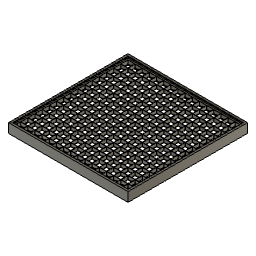
LED matrix v11 (Autodesk Fusion 360 design; units mm, degrees)
Autodesk Fusion 360 part; units mm, degrees
sketch "quad" plane through (0, 0, 0) normal (0, 0, 1) x (1, 0, 0)
  line L0 (0, 0) -> (10, 0)
  line L1 (10, 0) -> (10, 10)
  line L2 (10, 10) -> (0, 10)
  line L3 (0, 10) -> (0, 0)
  line L4 (9.75, 0.25) -> (9.75, 9.75)
  line L5 (9.75, 9.75) -> (0.25, 9.75)
  line L6 (0.25, 9.75) -> (0.25, 0.25)
  line L7 (0.25, 0.25) -> (9.75, 0.25)
  dimension "d1" = 10
  dimension "d2" = 10
  dimension "d3" = -0.25
  constraint horizontal L0
  constraint vertical L1
  constraint horizontal L2
  constraint vertical L3
  constraint coincident L0.start L3.end
  measures "d1" distance of L0.start L0.end
  measures "d2" distance of L0.start L2.end
extrude "Extrude1" add sketch "quad" along normal blind 5 makes body 1
sketch "hole" plane through (0, 0, 0) normal (0, 1, 0) x (1, 0, 0)
  line L0 (4.3, 0) -> (7.3, 0)
  line L1 (7.3, 0) -> (7.3, -0.5)
  line L2 (7, -0.8) -> (4.6, -0.8)
  line L3 (4.3, -0.5) -> (4.3, 0)
  arc A0 (4.3, -0.5) -> (4.6, -0.8) centre (4.6, -0.5) ccw
  arc A1 (7, -0.8) -> (7.3, -0.5) centre (7, -0.5) ccw
  point P0 (4.3, -0.8)
  point P1 (10, 0)
  dimension "d6" = 3
  dimension "d7" = 0.8
  dimension "d8" = 2.7
  dimension "d11" = 0.3
  dimension "d12" = 0.3
  constraint horizontal L0
  constraint vertical L1
  constraint horizontal L2
  constraint vertical L3
  constraint coincident P0 L2
  constraint coincident P0 L3
  constraint tangent L2 A0
  constraint tangent L3 A0
  constraint tangent L1 A1
  constraint tangent L2 A1
  measures "d6" distance of L0.start L0.end
  measures "d7" distance of L0.start P0
  measures "d8" distance of L0.end P1
  measures "d11" radius of A0
  measures "d12" radius of A1
extrude "Extrude2" cut sketch "hole" along normal blind 10 bodies 1
sketch "lid" plane through (0, 0, 5) normal (0, 0, 1) x (-1, 0, 0)
  line L0 (-9.75, -0.25) -> (-0.25, -0.25)
  line L1 (-0.25, -0.25) -> (-0.25, -9.75)
  line L2 (-0.25, -9.75) -> (-9.75, -9.75)
  line L3 (-9.75, -9.75) -> (-9.75, -0.25)
  line L4 (0, -10) -> (0, 0)
  line L5 (0, 0) -> (-10, 0)
  line L6 (-10, 0) -> (-10, -10)
  line L7 (-10, -10) -> (0, -10)
  line L8 (0, 0) -> (-10, 0)
  line L9 (-10, 0) -> (-10, -10)
  line L10 (-10, -10) -> (0, -10)
  line L11 (0, -10) -> (0, 0)
  constraint horizontal L8
  constraint vertical L9
  constraint horizontal L10
  constraint vertical L11
  constraint coincident L6.end L7.start
  constraint coincident L4.end L5.start
extrude "Extrude3" add sketch "lid" along normal blind 0.2 separate body contours L0 L1 L2 L3 | L4 L5 L6 L7 L8 L9 L10 L11 makes body 2
pattern_linear "R-Pattern1" count 16 spacing 10 along (0, 1, 0) count 16 spacing 10 along (1, 0, 0) of bodies 1 makes body 3 at (0, 16.6667, 1.6667) makes body 4 at (0, 26.6667, 1.6667) makes body 5 at (10, 6.6667, 1.6667) makes body 6 at (10.25, 16.5833, 1.6667) makes body 7 at (10.25, 26.5833, 1.6667) makes body 8 at (24.8667, 0, 3.6) makes body 9 at (20.25, 16.5833, 1.6667) makes body 10 at (20.25, 26.5833, 1.6667) makes body 11 at (0, 36.6667, 1.6667) makes body 12 at (0, 46.6667, 1.6667) makes body 13 at (0, 56.6667, 1.6667) makes body 14 at (0, 66.6667, 1.6667) makes body 15 at (0, 76.6667, 1.6667) makes body 16 at (0, 86.6667, 1.6667) makes body 17 at (0, 96.6667, 1.6667) makes body 18 at (0, 106.6667, 1.6667) makes body 19 at (0, 116.6667, 1.6667) makes body 20 at (0, 126.6667, 1.6667) makes body 21 at (0, 136.6667, 1.6667) makes body 22 at (0, 146.6667, 1.6667) makes body 23 at (0, 156.6667, 1.6667) makes body 24 at (10.25, 36.5833, 1.6667) makes body 25 at (10.25, 46.5833, 1.6667) makes body 26 at (10.25, 56.5833, 1.6667) makes body 27 at (10.25, 66.5833, 1.6667) makes body 28 at (10.25, 76.5833, 1.6667) makes body 29 at (10.25, 86.5833, 1.6667) makes body 30 at (10.25, 96.5833, 1.6667) makes body 31 at (10.25, 106.5833, 1.6667) makes body 32 at (10.25, 116.5833, 1.6667) makes body 33 at (10.25, 126.5833, 1.6667) makes body 34 at (10.25, 136.5833, 1.6667) makes body 35 at (10.25, 146.5833, 1.6667) makes body 36 at (14.8667, 160, 3.6) makes body 37 at (20.25, 36.5833, 1.6667) makes body 38 at (20.25, 46.5833, 1.6667) makes body 39 at (20.25, 56.5833, 1.6667) makes body 40 at (20.25, 66.5833, 1.6667) makes body 41 at (20.25, 76.5833, 1.6667) makes body 42 at (20.25, 86.5833, 1.6667) makes body 43 at (20.25, 96.5833, 1.6667) makes body 44 at (20.25, 106.5833, 1.6667) makes body 45 at (20.25, 116.5833, 1.6667) makes body 46 at (20.25, 126.5833, 1.6667) makes body 47 at (20.25, 136.5833, 1.6667) makes body 48 at (20.25, 146.5833, 1.6667) makes body 49 at (24.8667, 160, 3.6) makes body 50 at (34.8667, 0, 3.6) makes body 51 at (30.25, 16.5833, 1.6667) makes body 52 at (30.25, 26.5833, 1.6667) makes body 53 at (30.25, 36.5833, 1.6667) makes body 54 at (30.25, 46.5833, 1.6667) makes body 55 at (30.25, 56.5833, 1.6667) makes body 56 at (30.25, 66.5833, 1.6667) makes body 57 at (30.25, 76.5833, 1.6667) makes body 58 at (30.25, 86.5833, 1.6667) makes body 59 at (30.25, 96.5833, 1.6667) makes body 60 at (30.25, 106.5833, 1.6667) makes body 61 at (30.25, 116.5833, 1.6667) makes body 62 at (30.25, 126.5833, 1.6667) makes body 63 at (30.25, 136.5833, 1.6667) makes body 64 at (30.25, 146.5833, 1.6667) makes body 65 at (34.8667, 160, 3.6) makes body 66 at (44.8667, 0, 3.6) makes body 67 at (40.25, 16.5833, 1.6667) makes body 68 at (40.25, 26.5833, 1.6667) makes body 69 at (40.25, 36.5833, 1.6667) makes body 70 at (40.25, 46.5833, 1.6667) makes body 71 at (40.25, 56.5833, 1.6667) makes body 72 at (40.25, 66.5833, 1.6667) makes body 73 at (40.25, 76.5833, 1.6667) makes body 74 at (40.25, 86.5833, 1.6667) makes body 75 at (40.25, 96.5833, 1.6667) makes body 76 at (40.25, 106.5833, 1.6667) makes body 77 at (40.25, 116.5833, 1.6667) makes body 78 at (40.25, 126.5833, 1.6667) makes body 79 at (40.25, 136.5833, 1.6667) makes body 80 at (40.25, 146.5833, 1.6667) makes body 81 at (44.8667, 160, 3.6) makes body 82 at (54.8667, 0, 3.6) makes body 83 at (50.25, 16.5833, 1.6667) makes body 84 at (50.25, 26.5833, 1.6667) makes body 85 at (50.25, 36.5833, 1.6667) makes body 86 at (50.25, 46.5833, 1.6667) makes body 87 at (50.25, 56.5833, 1.6667) makes body 88 at (50.25, 66.5833, 1.6667) makes body 89 at (50.25, 76.5833, 1.6667) makes body 90 at (50.25, 86.5833, 1.6667) makes body 91 at (50.25, 96.5833, 1.6667) makes body 92 at (50.25, 106.5833, 1.6667) makes body 93 at (50.25, 116.5833, 1.6667) makes body 94 at (50.25, 126.5833, 1.6667) makes body 95 at (50.25, 136.5833, 1.6667) makes body 96 at (50.25, 146.5833, 1.6667) makes body 97 at (54.8667, 160, 3.6) makes body 98 at (64.8667, 0, 3.6) makes body 99 at (60.25, 16.5833, 1.6667) makes body 100 at (60.25, 26.5833, 1.6667) makes body 101 at (60.25, 36.5833, 1.6667) makes body 102 at (60.25, 46.5833, 1.6667) makes body 103 at (60.25, 56.5833, 1.6667) makes body 104 at (60.25, 66.5833, 1.6667) makes body 105 at (60.25, 76.5833, 1.6667) makes body 106 at (60.25, 86.5833, 1.6667) makes body 107 at (60.25, 96.5833, 1.6667) makes body 108 at (60.25, 106.5833, 1.6667) makes body 109 at (60.25, 116.5833, 1.6667) makes body 110 at (60.25, 126.5833, 1.6667) makes body 111 at (60.25, 136.5833, 1.6667) makes body 112 at (60.25, 146.5833, 1.6667) makes body 113 at (64.8667, 160, 3.6) makes body 114 at (74.8667, 0, 3.6) makes body 115 at (70.25, 16.5833, 1.6667) makes body 116 at (70.25, 26.5833, 1.6667) makes body 117 at (70.25, 36.5833, 1.6667) makes body 118 at (70.25, 46.5833, 1.6667) makes body 119 at (70.25, 56.5833, 1.6667) makes body 120 at (70.25, 66.5833, 1.6667) makes body 121 at (70.25, 76.5833, 1.6667) makes body 122 at (70.25, 86.5833, 1.6667) makes body 123 at (70.25, 96.5833, 1.6667) makes body 124 at (70.25, 106.5833, 1.6667) makes body 125 at (70.25, 116.5833, 1.6667) makes body 126 at (70.25, 126.5833, 1.6667) makes body 127 at (70.25, 136.5833, 1.6667) makes body 128 at (70.25, 146.5833, 1.6667) makes body 129 at (74.8667, 160, 3.6) makes body 130 at (84.8667, 0, 3.6) makes body 131 at (80.25, 16.5833, 1.6667) makes body 132 at (80.25, 26.5833, 1.6667) makes body 133 at (80.25, 36.5833, 1.6667) makes body 134 at (80.25, 46.5833, 1.6667) makes body 135 at (80.25, 56.5833, 1.6667) makes body 136 at (80.25, 66.5833, 1.6667) makes body 137 at (80.25, 76.5833, 1.6667) makes body 138 at (80.25, 86.5833, 1.6667) makes body 139 at (80.25, 96.5833, 1.6667) makes body 140 at (80.25, 106.5833, 1.6667) makes body 141 at (80.25, 116.5833, 1.6667) makes body 142 at (80.25, 126.5833, 1.6667) makes body 143 at (80.25, 136.5833, 1.6667) makes body 144 at (80.25, 146.5833, 1.6667) makes body 145 at (84.8667, 160, 3.6) makes body 146 at (94.8667, 0, 3.6) makes body 147 at (90.25, 16.5833, 1.6667) makes body 148 at (90.25, 26.5833, 1.6667) makes body 149 at (90.25, 36.5833, 1.6667) makes body 150 at (90.25, 46.5833, 1.6667) makes body 151 at (90.25, 56.5833, 1.6667) makes body 152 at (90.25, 66.5833, 1.6667) makes body 153 at (90.25, 76.5833, 1.6667) makes body 154 at (90.25, 86.5833, 1.6667) makes body 155 at (90.25, 96.5833, 1.6667) makes body 156 at (90.25, 106.5833, 1.6667) makes body 157 at (90.25, 116.5833, 1.6667) makes body 158 at (90.25, 126.5833, 1.6667) makes body 159 at (90.25, 136.5833, 1.6667) makes body 160 at (90.25, 146.5833, 1.6667) makes body 161 at (94.8667, 160, 3.6) makes body 162 at (104.8667, 0, 3.6) makes body 163 at (100.25, 16.5833, 1.6667) makes body 164 at (100.25, 26.5833, 1.6667) makes body 165 at (100.25, 36.5833, 1.6667) makes body 166 at (100.25, 46.5833, 1.6667) makes body 167 at (100.25, 56.5833, 1.6667) makes body 168 at (100.25, 66.5833, 1.6667) makes body 169 at (100.25, 76.5833, 1.6667) makes body 170 at (100.25, 86.5833, 1.6667) makes body 171 at (100.25, 96.5833, 1.6667) makes body 172 at (100.25, 106.5833, 1.6667) makes body 173 at (100.25, 116.5833, 1.6667) makes body 174 at (100.25, 126.5833, 1.6667) makes body 175 at (100.25, 136.5833, 1.6667) makes body 176 at (100.25, 146.5833, 1.6667) makes body 177 at (104.8667, 160, 3.6) makes body 178 at (114.8667, 0, 3.6) makes body 179 at (110.25, 16.5833, 1.6667) makes body 180 at (110.25, 26.5833, 1.6667) makes body 181 at (110.25, 36.5833, 1.6667) makes body 182 at (110.25, 46.5833, 1.6667) makes body 183 at (110.25, 56.5833, 1.6667) makes body 184 at (110.25, 66.5833, 1.6667) makes body 185 at (110.25, 76.5833, 1.6667) makes body 186 at (110.25, 86.5833, 1.6667) makes body 187 at (110.25, 96.5833, 1.6667) makes body 188 at (110.25, 106.5833, 1.6667) makes body 189 at (110.25, 116.5833, 1.6667) makes body 190 at (110.25, 126.5833, 1.6667) makes body 191 at (110.25, 136.5833, 1.6667) makes body 192 at (110.25, 146.5833, 1.6667) makes body 193 at (114.8667, 160, 3.6) makes body 194 at (124.8667, 0, 3.6) makes body 195 at (120.25, 16.5833, 1.6667) makes body 196 at (120.25, 26.5833, 1.6667) makes body 197 at (120.25, 36.5833, 1.6667) makes body 198 at (120.25, 46.5833, 1.6667) makes body 199 at (120.25, 56.5833, 1.6667) makes body 200 at (120.25, 66.5833, 1.6667) makes body 201 at (120.25, 76.5833, 1.6667) makes body 202 at (120.25, 86.5833, 1.6667) makes body 203 at (120.25, 96.5833, 1.6667) makes body 204 at (120.25, 106.5833, 1.6667) makes body 205 at (120.25, 116.5833, 1.6667) makes body 206 at (120.25, 126.5833, 1.6667) makes body 207 at (120.25, 136.5833, 1.6667) makes body 208 at (120.25, 146.5833, 1.6667) makes body 209 at (124.8667, 160, 3.6) makes body 210 at (134.8667, 0, 3.6) makes body 211 at (130.25, 16.5833, 1.6667) makes body 212 at (130.25, 26.5833, 1.6667) makes body 213 at (130.25, 36.5833, 1.6667) makes body 214 at (130.25, 46.5833, 1.6667) makes body 215 at (130.25, 56.5833, 1.6667) makes body 216 at (130.25, 66.5833, 1.6667) makes body 217 at (130.25, 76.5833, 1.6667) makes body 218 at (130.25, 86.5833, 1.6667) makes body 219 at (130.25, 96.5833, 1.6667) makes body 220 at (130.25, 106.5833, 1.6667) makes body 221 at (130.25, 116.5833, 1.6667) makes body 222 at (130.25, 126.5833, 1.6667) makes body 223 at (130.25, 136.5833, 1.6667) makes body 224 at (130.25, 146.5833, 1.6667) makes body 225 at (134.8667, 160, 3.6) makes body 226 at (144.8667, 0, 3.6) makes body 227 at (140.25, 16.5833, 1.6667) makes body 228 at (140.25, 26.5833, 1.6667) makes body 229 at (140.25, 36.5833, 1.6667) makes body 230 at (140.25, 46.5833, 1.6667) makes body 231 at (140.25, 56.5833, 1.6667) makes body 232 at (140.25, 66.5833, 1.6667) makes body 233 at (140.25, 76.5833, 1.6667) makes body 234 at (140.25, 86.5833, 1.6667) makes body 235 at (140.25, 96.5833, 1.6667) makes body 236 at (140.25, 106.5833, 1.6667) makes body 237 at (140.25, 116.5833, 1.6667) makes body 238 at (140.25, 126.5833, 1.6667) makes body 239 at (140.25, 136.5833, 1.6667) makes body 240 at (140.25, 146.5833, 1.6667) makes body 241 at (144.8667, 160, 3.6) makes body 242 at (160, 3.3333, 1.6667) makes body 243 at (160, 13.3333, 1.6667) makes body 244 at (160, 23.3333, 1.6667) makes body 245 at (160, 33.3333, 1.6667) makes body 246 at (160, 43.3333, 1.6667) makes body 247 at (160, 53.3333, 1.6667) makes body 248 at (160, 63.3333, 1.6667) makes body 249 at (160, 73.3333, 1.6667) makes body 250 at (160, 83.3333, 1.6667) makes body 251 at (160, 93.3333, 1.6667) makes body 252 at (160, 103.3333, 1.6667) makes body 253 at (160, 113.3333, 1.6667) makes body 254 at (160, 123.3333, 1.6667) makes body 255 at (160, 133.3333, 1.6667) makes body 256 at (160, 143.3333, 1.6667) makes body 257 at (160, 153.3333, 1.6667)
sketch "frame" plane through (0, 0, 0) normal (0, 0, 1) x (1, 0, 0)
  line L0 (0, 0) -> (160, 0)
  line L1 (160, 0) -> (160, 160)
  line L2 (160, 160) -> (0, 160)
  line L3 (0, 160) -> (0, 0)
  line L4 (162, 162) -> (-2, 162)
  line L5 (-2, 162) -> (-2, -2)
  line L6 (-2, -2) -> (162, -2)
  line L7 (162, -2) -> (162, 162)
  line L8 (-3.5, 163.5) -> (-3.5, -3.5)
  line L9 (-3.5, -3.5) -> (163.5, -3.5)
  line L10 (163.5, -3.5) -> (163.5, 163.5)
  line L11 (163.5, 163.5) -> (-3.5, 163.5)
  line L12 (160.5, -0.5) -> (160.5, 160.5)
  line L13 (160.5, 160.5) -> (-0.5, 160.5)
  line L14 (-0.5, 160.5) -> (-0.5, -0.5)
  line L15 (-0.5, -0.5) -> (160.5, -0.5)
  line L16 (162.5, -2.5) -> (162.5, 162.5)
  line L17 (162.5, 162.5) -> (-2.5, 162.5)
  line L18 (-2.5, 162.5) -> (-2.5, -2.5)
  line L19 (-2.5, -2.5) -> (162.5, -2.5)
  dimension "d41" = 160
  dimension "d42" = 160
  dimension "d43" = 2
  dimension "d44" = 3.5
  dimension "d50" = 0.5
  dimension "d59" = 2.5
  constraint horizontal L0
  constraint vertical L1
  constraint horizontal L2
  constraint vertical L3
  constraint coincident L0.start L3.end
  measures "d41" distance of L0.start L0.end
  measures "d42" distance of L0.start L2.end
extrude "Extrude4" add sketch "frame" along normal blind 5 separate body contours L4 L5 L6 L7 | L12 L13 L14 L15 makes body 258
extrude "Extrude9" add sketch "frame" against normal blind 1.5 contours L4 L5 L6 L7 bodies 258
extrude "Extrude6" add sketch "frame" along normal blind 8 and the other way blind 4 separate body contours L8 L9 L10 L11 makes body 259
sketch "lid frame" plane through (0, 0, 8) normal (0, 0, 1) x (-1, 0, 0)
  line L0 (-163.5, -163.5) -> (3.5, -163.5)
  line L1 (3.5, -163.5) -> (3.5, 3.5)
  line L2 (3.5, 3.5) -> (-163.5, 3.5)
  line L3 (-163.5, 3.5) -> (-163.5, -163.5)
  line L4 (-162.5, 2.5) -> (2.5, 2.5)
  line L5 (2.5, 2.5) -> (2.5, -162.5)
  line L6 (2.5, -162.5) -> (-162.5, -162.5)
  line L7 (-162.5, -162.5) -> (-162.5, 2.5)
  line L8 (-160.5, -160.5) -> (-160.5, 0.5)
  line L9 (-160.5, 0.5) -> (0.5, 0.5)
  line L10 (0.5, 0.5) -> (0.5, -160.5)
  line L11 (0.5, -160.5) -> (-160.5, -160.5)
  dimension "d68" = 2
extrude "Extrude7" add sketch "lid frame" along normal blind 1 contours L0 L1 L2 L3 | L4 L5 L6 L7 bodies 259
sketch "PCB hooks" plane through (160.5, 0, 0) normal (-1, 0, 0) x (0, 1, 0)
  line L0 (160, 5) -> (0, 5)
  line L1 (0, 5) -> (0, 0)
  line L2 (0, 0) -> (160, 0)
  line L3 (160, 0) -> (160, 5)
  line L4 (162, -1.5) -> (162, 5)
  line L5 (162, 5) -> (-2, 5)
  line L6 (-2, 5) -> (-2, -1.5)
  line L7 (-2, -1.5) -> (162, -1.5)
  line L8 (-0.5, 0) -> (160.5, 0)
  line L9 (160.5, 0) -> (160.5, 1.5)
  line L10 (160.5, 1.5) -> (-0.5, 1.5)
  line L11 (-0.5, 1.5) -> (-0.5, 0)
  line L12 (3, 1.5) -> (7, 1.5)
  line L13 (7, 1.5) -> (7, 0.5)
  line L14 (7, 0.5) -> (3, 0.5)
  line L15 (3, 0.5) -> (3, 1.5)
  dimension "d53" = 4
  dimension "d54" = 1
  dimension "d55" = 3
  constraint horizontal L12
  constraint vertical L13
  constraint horizontal L14
  constraint vertical L15
  constraint coincident L10 L12.start
  measures "d53" distance of L12.start L12.end
  measures "d54" distance of L12.start L14.end
  measures "d55" distance of L1 L15
extrude "Extrude8" add sketch "PCB hooks" along normal blind 1 separate body contours L10 L12 L13 L14 L15 makes body 260
extrude "Extrude10" add sketch "PCB hooks" against normal blind 1 from surface at 161 separate body contours L10 L12 L13 L14 L15 makes body 261
pattern_linear "R-Pattern2" count 3 spacing 75 along (0, 1, 0) of bodies 261 260 makes body 262 at (160.5, 79.3333, -1.1667) makes body 263 at (160.5, 154.3333, -0.8333) makes body 264 at (-0.5, 79.3333, -1.1667) makes body 265 at (-0.5, 154.3333, -0.8333)
copy_body "CopyPasteBodies2" bodies 260 makes body 266
move_body "Move2" bodies 266 to x (0, 1, 0) y (-1, 0, 0) z (0, 0, 1) at (160, -160, 0)
copy_body "CopyPasteBodies3" bodies 266 makes body 267
move_body "Move3" bodies 267 to x (1, 0, 0) y (0, 1, 0) z (0, 0, 1) at (0, 160, 0)
pattern_linear "R-Pattern3" count 3 spacing 75 along (-1, 0, 0) of bodies 266 267 makes body 268 at (80.6667, 0.5, -1.1667) makes body 269 at (5.6667, 0.5, -1.1667) makes body 270 at (80.6667, 160.5, -1.1667) makes body 271 at (5.6667, 160.5, -1.1667)
hidden bodies 2
equation "h = 5 mm"
equation "d20 = h"
equation "d28 = h + 3 mm"
equation "d48 = -( 160 mm - 3 mm - 4 mm - 3 mm )"
equation "d66 = 160 mm - ( 2 * 3 ) * 1 mm - 4 mm"
named bodies: "box", "lid", "box (1)", "box (2)", "box (3)", "box (4)", "box (5)", "box (6)", "box (7)", "box (8)", "frame grid", "frame lid", "PCB hook 1", "PCB hook (1)", "PCB hook (2)", "box (9)", "box (10)", "box (11)", "box (12)", "box (13)", "box (14)", "box (15)", "box (16)", "box (17)", "box (18)", "box (19)", "box (20)", "box (21)", "box (22)", "box (23)", "box (24)", "box (25)", "box (26)", "box (27)", "box (28)", "box (29)", "box (30)", "box (31)", "box (32)", "box (33)", "box (34)", "box (35)", "box (36)", "box (37)", "box (38)", "box (39)", "box (40)", "box (41)", "box (42)", "box (43)", "box (44)", "box (45)", "box (46)", "box (47)", "box (48)", "box (49)", "box (50)", "box (51)", "box (52)", "box (53)", "box (54)", "box (55)", "box (56)", "box (57)", "box (58)", "box (59)", "box (60)", "box (61)", "box (62)", "box (63)", "box (64)", "box (65)", "box (66)", "box (67)", "box (68)", "box (69)", "box (70)", "box (71)", "box (72)", "box (73)", "box (74)", "box (75)", "box (76)", "box (77)", "box (78)", "box (79)", "box (80)", "box (81)", "box (82)", "box (83)", "box (84)", "box (85)", "box (86)", "box (87)", "box (88)", "box (89)", "box (90)", "box (91)", "box (92)", "box (93)", "box (94)", "box (95)", "box (96)", "box (97)", "box (98)", "box (99)", "box (100)", "box (101)", "box (102)", "box (103)", "box (104)", "box (105)", "box (106)", "box (107)", "box (108)", "box (109)", "box (110)", "box (111)", "box (112)", "box (113)", "box (114)", "box (115)", "box (116)", "box (117)", "box (118)", "box (119)", "box (120)", "box (121)", "box (122)", "box (123)", "box (124)", "box (125)", "box (126)", "box (127)", "box (128)", "box (129)", "box (130)", "box (131)", "box (132)", "box (133)", "box (134)", "box (135)", "box (136)", "box (137)", "box (138)", "box (139)", "box (140)", "box (141)", "box (142)", "box (143)", "box (144)", "box (145)", "box (146)", "box (147)", "box (148)", "box (149)", "box (150)", "box (151)", "box (152)", "box (153)", "box (154)", "box (155)", "box (156)", "box (157)", "box (158)", "box (159)", "box (160)", "box (161)", "box (162)", "box (163)", "box (164)", "box (165)", "box (166)", "box (167)", "box (168)", "box (169)", "box (170)", "box (171)", "box (172)", "box (173)", "box (174)", "box (175)", "box (176)", "box (177)", "box (178)", "box (179)", "box (180)", "box (181)", "box (182)", "box (183)", "box (184)", "box (185)", "box (186)", "box (187)", "box (188)", "box (189)", "box (190)", "box (191)", "box (192)", "box (193)", "box (194)", "box (195)", "box (196)", "box (197)", "box (198)", "box (199)", "box (200)", "box (201)", "box (202)", "box (203)", "box (204)", "box (205)", "box (206)", "box (207)", "box (208)", "box (209)", "box (210)", "box (211)", "box (212)", "box (213)", "box (214)", "box (215)", "box (216)", "box (217)", "box (218)", "box (219)", "box (220)", "box (221)", "box (222)", "box (223)", "box (224)", "box (225)", "box (226)", "box (227)", "box (228)", "box (229)", "box (230)", "box (231)", "box (232)", "box (233)", "box (234)", "box (235)", "box (236)", "box (237)", "box (238)", "box (239)", "box (240)", "box (241)", "box (242)", "box (243)", "box (244)", "box (245)", "box (246)", "box (247)", "box (248)", "box (249)", "box (250)", "box (251)", "box (252)", "box (253)", "box (254)", "box (255)", "PCB hook 2", "PCB hook 2 (1)", "PCB hook 2 (2)", "PCB hook 1 (1)", "PCB hook 1 (1) (1)", "PCB hook 1 (1) (2)", "PCB hook 1 (1) (3)", "PCB hook 1 (1) (1) (1)", "PCB hook 1 (1) (1) (2)"
